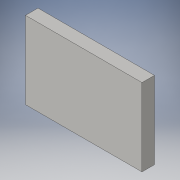
# Autodesk Inventor part: mcdave_breadboard
Saved by Autodesk Inventor 2016 (Build 200138000, 138)
## iProperties
Created: 2017-09-08
Part Number: mcdave_breadboard
Material: Generic
Document SubType Name: Modeling
Designer: student
Density: 1 g/cm^3
Appearance: Default
Author: student
Autodesk Inventor part; units mm, degrees
ref_plane "YZ Plane" through (0, 0, 0) normal (1, 0, 0) x (0, 1, 0)
ref_plane "XZ Plane" through (0, 0, 0) normal (0, 1, 0) x (-1, 0, 0)
ref_plane "XY Plane" through (0, 0, 0) normal (0, 0, 1) x (1, 0, 0)
sketch "Sketch1" plane through (0, 0, 0) normal (0, 0, 1) x (1, 0, 0)
  line L0 (11.1364, 3.5202) -> (51.8653, 3.5202)
  line L1 (51.8653, 3.5202) -> (51.8653, -50.5818)
  line L2 (51.8653, -50.5818) -> (11.1364, -50.5818)
  line L3 (11.1364, -50.5818) -> (-29.5925, -50.5818)
  line L4 (11.1364, 3.5202) -> (-29.5925, 3.5202)
  line L5 (-29.5925, 3.5202) -> (-29.5925, -50.5818)
  line L6 (51.8653, 3.5202) -> (-29.5925, 3.5202)
  line L7 (-29.5925, 3.5202) -> (-29.5925, -50.5818)
  line L8 (51.8653, -50.5818) -> (-29.5925, -50.5818)
  line L9 (51.8653, -50.5818) -> (51.8653, 3.5202)
  point P0 (0, 0)
  point P1 (0, 0)
  dimension "d0" = 40.7289
  dimension "d1" = 40.7289
  constraints: 20 end point, 4 collinear, 2 horizontal, 1 point on line, 1 vertical
  measures "d0" distance of L0.start L0.end
  measures "d1" distance of L2.end L3.end
extrude "Extrusion1" add sketch "Sketch1" along normal blind 8.7376
body "Solid1"
